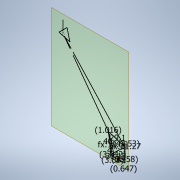
# Autodesk Inventor part: PrismsGeometry
Saved by Autodesk Inventor 2020 (Build 240168000, 168)
## iProperties
Created: 2017-01-26
Part Number: PrismsGeometry
Material: Nylon 6/6
Document SubType Name: Modeling
Designer: vmigu
Density: 1.13 g/cm^3
Appearance: Tropical Blue
Mass: 88.1271 g
Surface Area: 339.5 cm^2
Volume: 77.9886 cm^3
Author: vmigu
Autodesk Inventor part; units mm, degrees
ref_plane "YZ Plane" through (0, 0, 0) normal (1, 0, 0) x (0, 1, 0)
ref_plane "XZ Plane" through (0, 0, 0) normal (0, 1, 0) x (-1, 0, 0)
ref_plane "XY Plane" through (0, 0, 0) normal (0, 0, 1) x (1, 0, 0)
sketch "PENTAPRISMA" plane through (0, 0, 0) normal (0, 0, 1) x (1, 0, 0)
  line L0 (-36.8404, 92.0637) -> (-26.2338, 81.4571)
  line L1 (-26.2338, 81.4571) -> (-15.6272, 92.0637)
  line L2 (-15.6272, 92.0637) -> (-20.5273, 103.8937)
  line L3 (-20.5273, 103.8937) -> (-31.9403, 103.8937)
  line L4 (-31.9403, 103.8937) -> (-36.8404, 92.0637)
  line L5 (-20.9305, 86.7604) -> (-26.2338, 92.0637) construction
  line L6 (-26.2338, 92.0637) -> (-31.5371, 86.7604) construction
  line L7 (-26.2338, 81.4571) -> (-26.2338, 103.8937) construction
  dimension "d114" = 90
  dimension "d115" = 112.5
  dimension "d116" = 112.5
  dimension "d117" = 112.5
  dimension "d118" = 15
  measures "d114" angle of L0 L1
  measures "d115" angle of L2 L1
  measures "d116" angle of L2 L3
  measures "d117" angle of L0 L4
  measures "d118" distance of L1.start L1.end
sketch "PRISMA.ENTRADA" plane through (0, 0, 0) normal (0, 0, 1) x (1, 0, 0)
  line L0 (57.6201, 1.807) -> (40.3499, 20.4323)
  line L1 (40.3499, 20.4323) -> (32.8551, -3.8368)
  line L2 (32.8551, -3.8368) -> (57.6201, 1.807)
  line L3 (45.2376, -1.0149) -> (46.3486, -5.8899) construction
  line L4 (45.2376, -1.0149) -> (62.1685, -11.6611)
  line L5 (45.2376, -1.0149) -> (37.1097, 9.9401) construction
  line L6 (45.2376, -1.0149) -> (36.8424, 9.0746) construction
  line L7 (37.1097, 9.9401) -> (31.8295, 29.2305)
  line L8 (36.8424, 9.0746) -> (29.4513, 27.6587)
  line L9 (45.2376, -1.0149) -> (35.5983, 5.0463) construction
  point P0 (40.854, 14.8365)
  dimension "d132" = 5
  dimension "d133" = 25.4
  dimension "d134" = 20
  dimension "d135" = 45
  dimension "d136" = 20
  dimension "d137" = 20
  dimension "d140" = 42.53
  dimension "d141" = 36.15
  dimension "d142" = 18.075
  dimension "d143" = 21.265
  measures "d132" distance of L9.start L3.end
  measures "d133" distance of L1.end L2.end
  measures "d134" distance of L9.start L4.end
  measures "d135" angle of L4 L3
  measures "d136" distance of L5.end L7.end
  measures "d137" distance of L6.end L8.end
  measures "d140" angle of L7 L9
  measures "d141" angle of L9 L8
  measures "d142" angle of L9 L6
  measures "d143" angle of L9 L5
sketch "OTICA" plane through (0, 0, 0) normal (0, 1, 0) x (-1, 0, 0)
  line L0 (23.4165, 43.0473) -> (14.7385, 4)
  line L1 (14.7385, 4) -> (-14.7385, 31.039)
  line L2 (-14.7385, 31.039) -> (23.4165, 43.0473)
  line L3 (7.0299, 37.8901) -> (22.401, 42.7277) construction
  line L4 (101.5992, 157.0905) -> (-13.7385, 31.3538)
  line L5 (101.6654, 151.2273) -> (22.401, 42.7277)
  line L6 (14.55, 0) -> (-14.55, 0)
  line L7 (-13.7385, 31.3538) -> (-14.3522, 30.6847) construction
  line L8 (22.401, 42.7277) -> (2.3861, 15.3307) construction
  line L9 (22.401, 42.7277) -> (10.9082, 7.5135)
  line L10 (10.9082, 7.5135) -> (10.9082, 0)
  line L11 (-13.7385, 31.3538) -> (-14.0918, 30.4459)
  line L12 (-14.0918, 30.4459) -> (-14.0918, 0)
  line L13 (14.55, 0) -> (14.55, 4)
  line L14 (14.55, 4) -> (14.7385, 4)
  line L15 (-14.55, 0) -> (-14.55, 31.039)
  line L16 (-14.55, 31.039) -> (-14.7385, 31.039)
  line L17 (14.55, 0) -> (55.2636, 0)
  line L18 (115.4746, 198.3059) -> (108.9006, 173.7714)
  line L19 (108.9006, 173.7714) -> (133.4351, 180.3454)
  line L20 (133.4351, 180.3454) -> (115.4746, 198.3059)
  line L21 (124.4548, 189.3256) -> (127.9904, 192.8612) construction
  line L22 (124.4548, 189.3256) -> (124.4548, 209.3256)
  line L23 (124.4548, 189.3256) -> (119.5075, 176.6135) construction
  line L24 (124.4548, 189.3256) -> (120.3825, 176.8479) construction
  line L25 (119.5075, 176.6135) -> (105.988, 161.875)
  line L26 (120.3825, 176.8479) -> (108.5845, 160.6984)
  line L27 (124.4548, 189.3256) -> (124.4548, 177.9391) construction
  point P0 (0, 0)
  point P1 (0, 0)
  point P2 (0, 0)
  point P3 (-14.55, 30.8662)
  dimension "d1" = 40
  dimension "d188" = 29.1
  dimension "d189" = 36.15
  dimension "d190" = 42.53
  dimension "d191" = 21.265
  dimension "d192" = 18.075
  dimension "d197" = 4
  dimension "d205" = 1
  dimension "d208" = 25
  dimension "d209" = 0.4582
  dimension "d210" = 3.6418
  dimension "d211" = 1.0155
  dimension "d212" = 0.6467
  dimension "d213" = 3.8303
  constraints: 36 end point, 9 point on line, 5 perpendicular, 3 equal length, 2 coincident, 2 collinear, 2 horizontal, 2 vertical, 1 midpoint, 2 other
  measures "d1" distance of L0.start L0.end
  measures "d188" distance of L6.start L6.end
  measures "d189" angle of L10 L8
  measures "d190" angle of L12 L4
  measures "d191" angle of L11 L7
  measures "d192" angle of L8 L9
  measures "d197" distance of L6.start L13.end
  measures "d205" horizontal distance of L4.end L1.end
  measures "d208" distance between parallel lines of L10 L12
  measures "d209" distance from line of L6.end L12
  measures "d210" distance between parallel lines of L13 L10
  measures "d211" horizontal distance of L3.end L0.start
  measures "d212" distance from line of L12 L1.end
  measures "d213" distance from line of L0.end L10
extrude "Extrusion20" add sketch "OTICA" along normal mid plane 25.4 contours L20 L19 L18
extrude "Extrusion21" add sketch "OTICA" along normal mid plane 20 contours L0 L1 L9 L2 | L9 L1 L11 L2 | L11 L1 L15 L16 L2
body "Solid5"
